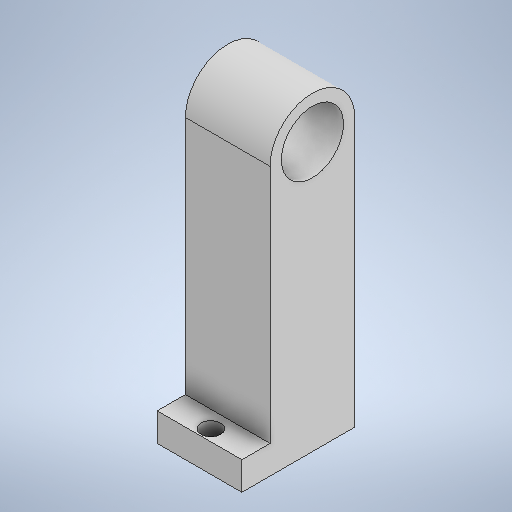
# Autodesk Inventor part: Holder_slim_1_fod_venstre
Saved by Autodesk Inventor 2025.2 (Build 292293000, 293)
## iProperties
Created: 2025-05-06
Part Number: Holder_slim_1_fod_venstre
Material: Generic
Document SubType Name: Modeling
Designer: lauri
Density: 1 g/cm^3
Appearance: Default
Author: lauri
Autodesk Inventor part; units mm, degrees
ref_plane "YZ Plane" through (0, 0, 0) normal (1, 0, 0) x (0, 1, 0)
ref_plane "XZ Plane" through (0, 0, 0) normal (0, 1, 0) x (-1, 0, 0)
ref_plane "XY Plane" through (0, 0, 0) normal (0, 0, 1) x (1, 0, 0)
sketch "Sketch1" plane through (0, 0, 0) normal (0, 1, 0) x (-1, 0, 0)
  line L0 (7.5, 12.5) -> (-7.5, 12.5)
  line L1 (-7.5, 12.5) -> (-7.5, -12.5)
  line L2 (-7.5, -12.5) -> (7.5, -12.5)
  line L3 (7.5, -12.5) -> (7.5, 12.5)
  line L4 (7.5, 12.5) -> (-7.5, -12.5) construction
  line L5 (-7.5, 12.5) -> (7.5, -12.5) construction
  point P0 (0, 0)
  dimension "d0" = 15
  dimension "d1" = 25
  constraints: 12 end point, 2 midpoint, 2 parallel, 1 horizontal, 1 perpendicular
  measures "d0" distance of L2.end L1.end
  measures "d1" distance of L1.end L0.end
extrude "Extrusion1" add sketch "Sketch1" along normal blind 5
sketch "Sketch2" plane through (0, 5, 0) normal (0, 1, 0) x (1, 0, 0)
  line L0 (-7.5, -12.5) -> (7.5, -12.5) projected
  line L1 (-7.5, 12.5) -> (-7.5, -12.5) projected
  line L2 (7.5, 7.5) -> (-7.5, 7.5)
  line L3 (-7.5, 7.5) -> (-7.5, -7.5)
  line L4 (-7.5, -7.5) -> (7.5, -7.5)
  line L5 (7.5, -7.5) -> (7.5, 7.5)
  line L6 (7.5, 7.5) -> (-7.5, -7.5) construction
  line L7 (-7.5, 7.5) -> (7.5, -7.5) construction
  point P0 (0, 0)
  dimension "d5" = 15
  constraints: 12 end point, 2 midpoint, 2 parallel, 1 horizontal, 1 perpendicular, 1 point on line
  measures "d5" distance of L3.end L2.end
extrude "Extrusion2" add sketch "Sketch2" along normal blind 50
sketch "Sketch3" plane through (7.5, 0, 12.5) normal (1, 0, 0) x (0, 0, -1)
  circle A0 centre (12.5, 47.5) radius 5.5
  point P0 (12.5, 0)
  point P1 (14.5, 47.5)
  dimension "d9" = 11
  constraints: 4 coincident, 1 centre point
  measures "d9" diameter of A0
extrude "Extrusion3" cut sketch "Sketch3" against normal blind 13
fillet "Fillet1" radius 7.5 2 edges at (0, 55, -7.5) (0, 55, 7.5)
sketch "Sketch5" plane through (0, 5, 0) normal (0, 1, 0) x (1, 0, 0)
  line L0 (7.5, -7.5) -> (-7.5, -7.5) projected
  line L1 (-7.5, -12.5) -> (7.5, -12.5) projected
  line L2 (-7.5, 7.5) -> (7.5, 7.5) projected
  line L3 (7.5, 12.5) -> (-7.5, 12.5) projected
  point P0 (0, 0)
  point P1 (0, -10.5)
  point P2 (0, 10.5)
hole "Hole2" at (0, 5, 10.5) at (0, 5, -10.5) direction (0, -1, 0) diameter 3.5 end through all
sketch "Sketch6" plane through (0, 5, 0) normal (0, 1, 0) x (1, 0, 0)
  point P0 (0, 0)
sketch "Sketch8" plane through (0, 5, 0) normal (0, 1, 0) x (1, 0, 0)
  line L0 (-7.5, 12.5) -> (-7.5, 7.5) projected
  line L1 (7.5, 12.5) -> (-7.5, 12.5) projected
  line L2 (-7.5, 7.5) -> (7.5, 7.5)
  line L3 (7.5, 7.5) -> (7.5, 12.5)
  line L4 (7.5, 12.5) -> (-7.5, 12.5)
  line L5 (-7.5, 12.5) -> (-7.5, 7.5)
  point P0 (0, 0)
  constraints: 8 end point, 2 parallel, 1 horizontal, 1 perpendicular
extrude "Extrusion5" cut sketch "Sketch8" against normal through all
body "Solid1"
